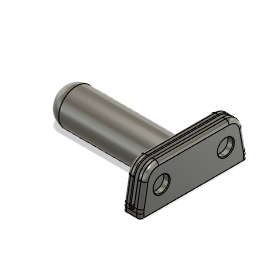
One Piece Handle v3 (Autodesk Fusion 360 design; units mm, degrees)
Autodesk Fusion 360 part; units mm, degrees
note: some values were not read from the file. Chosen so that the rebuilt part matches the saved one: which pieces of a blend or face edit are solid. Set by a fixed rule: which sketch regions a step uses.
sketch "Sketch1" plane through (0, 0, 0) normal (1, 0, 0) x (0, 0, -1)
  line L0 (-37.5, 0) -> (-33.0918, 25)
  line L1 (-33.0918, 25) -> (33.0918, 25)
  line L2 (33.0918, 25) -> (37.5, 0)
  line L3 (37.5, 0) -> (-37.5, 0)
  line L4 (0, 0) -> (0, 25) construction
  dimension "d2" = 75
  dimension "d3" = 80
  dimension "d5" = 100
  dimension "d6" = 25
  constraint horizontal L1
  constraint parallel L1 L3
  constraint coincident L4.start origin
  constraint midpoint L1 L4.end
  constraint vertical L4
  constraint coincident L4.start L3
  measures "d2" distance of L0.start L2.end
  measures "d3" angle of L2 L3
  measures "d5" angle of L0 L3
  measures "d6" distance of L1 L3
extrude "Extrude1" add sketch "Sketch1" along normal blind 5 from surface at 1.125 makes body 1
extrude "Extrude2" add sketch "Sketch1" against normal blind 5 from surface at -1.125 separate body makes body 2
sketch "Sketch2" plane through (0, 0, 0) normal (0, -1, 0) x (1, 0, 0)
  line L0 (1.125, 37.5) -> (1.125, -37.5)
  line L1 (1.125, -37.5) -> (6.125, -37.5)
  line L2 (6.125, -37.5) -> (6.125, 37.5)
  line L3 (6.125, 37.5) -> (1.125, 37.5)
  line L4 (6.125, 37.5) -> (-6.125, 37.5)
  line L5 (-6.125, 37.5) -> (-6.125, -37.5)
  line L6 (-6.125, -37.5) -> (6.125, -37.5)
  line L7 (6.125, -37.5) -> (6.125, 37.5)
  dimension "d13" = 12.25
  dimension "d14" = 75
  constraint horizontal L4
  constraint vertical L5
  constraint horizontal L6
  constraint vertical L7
  constraint coincident L2.end L3.start
  measures "d13" distance of L2.end L4.end
  measures "d14" distance of L2.end L1.end
extrude "Extrude3" add sketch "Sketch2" along normal blind 5 bodies 1 2
sketch "Sketch3" plane through (-6.125, 0, 0) normal (-1, 0, 0) x (0, 0, 1)
  line L0 (-33.0918, 25) -> (-37.5, 0)
  line L1 (-37.5, 0) -> (-37.5, -5)
  line L2 (-37.5, -5) -> (37.5, -5)
  line L3 (37.5, -5) -> (37.5, 0)
  line L4 (37.5, 0) -> (33.0918, 25)
  line L5 (33.0918, 25) -> (-33.0918, 25)
  line L6 (0, -5) -> (0, 5) construction
  circle A0 centre (0, 5) radius 12.5
  dimension "d17" = 25
  dimension "d18" = 10
  constraint midpoint L2 L6.start
  constraint perpendicular L2 L6
  constraint coincident L6.end A0.centre
  measures "d17" diameter of A0
  measures "d18" distance of L6.start L6.end
extrude "Extrude4" add sketch "Sketch3" along normal blind 80 contours L2 A0 picked at (0.0683, 3.2087) bodies 1
fillet "Fillet1" radius 10 1 edges at (-86.125, 17.5, 0) on bodies 1
fillet "Fillet2" radius 10 4 edges at (3.625, 25, 33.0918) (-3.625, 25, 33.0918) (-3.625, 25, -33.0918) (3.625, 25, -33.0918) on bodies 1
fillet "Fillet3" radius 15 4 edges at (3.625, 0, 37.5) (-3.625, 0, 37.5) (-3.625, 0, -37.5) (3.625, 0, -37.5) on bodies 1
fillet "Fillet4" radius 2.5 18 edges at (-6.125, -3.1562, -37.5) (-6.125, -0.005, -37.4429) (-6.125, 9.0144, -35.9105) (-6.125, 22.6604, -31.1287) (-6.125, 25, 0) (-6.125, 22.6604, 31.1287) (-6.125, 9.0144, 35.9105) (-6.125, -0.005, 37.4429) (-6.125, -3.1562, 37.5) (6.125, -3.1562, 37.5) (6.125, -0.005, 37.4429) (6.125, 9.0144, 35.9105) (6.125, 22.6604, 31.1287) (6.125, 25, 0) (6.125, 22.6604, -31.1287) (6.125, 9.0144, -35.9105) (6.125, -0.005, -37.4429) (6.125, -3.1562, -37.5) on bodies 1
chamfer "Chamfer1" distance 1 angle 45 12 edges at (-41.125, -5, 7.5) (-82.7394, -5, 0) (-41.125, -5, -7.5) (-6.125, -5, 21.25) (-6.125, -5, -21.25) (-5.3928, -5, -36.7678) (0, -5, -37.5) (5.3928, -5, -36.7678) (6.125, -5, 0) (5.3928, -5, 36.7678) (0, -5, 37.5) (-5.3928, -5, 36.7678) on bodies 1
sketch "Sketch4" plane through (-6.125, 0, 0) normal (-1, 0, 0) x (0, 0, 1)
  line L0 (8.6747, -4) -> (35, -4)
  line L1 (35, -4) -> (35, -1.3123)
  arc A0 (35, -1.3123) -> (34.8101, 0.8583) centre (22.5, -1.3123) ccw
  line L2 (34.8101, 0.8583) -> (32.0869, 16.3024)
  arc A1 (32.0869, 16.3024) -> (24.7008, 22.5) centre (24.7008, 15) ccw
  line L3 (24.7008, 22.5) -> (-24.7008, 22.5)
  arc A2 (-24.7008, 22.5) -> (-32.0869, 16.3024) centre (-24.7008, 15) ccw
  line L4 (-32.0869, 16.3024) -> (-34.8101, 0.8583)
  arc A3 (-34.8101, 0.8583) -> (-35, -1.3123) centre (-22.5, -1.3123) ccw
  line L5 (-35, -1.3123) -> (-35, -4)
  line L6 (-35, -4) -> (-8.6747, -4)
  arc A4 (8.6747, -4) -> (-8.6747, -4) centre (0, 5) ccw
  circle A5 centre (-22.5, 10) radius 5.5
  circle A6 centre (22.5, 10) radius 5.5
  dimension "d30" = 11
  dimension "d31" = 11
  dimension "d32" = 45
  dimension "d33" = 10
  dimension "d34" = 22.5
  constraint horizontal A5.centre A6.centre
  measures "d30" diameter of A5
  measures "d31" diameter of A6
  measures "d32" horizontal distance of A5.centre A6.centre
  measures "d33" vertical distance of origin A5.centre
  measures "d34" horizontal distance of origin A5.centre
extrude "Extrude5" cut sketch "Sketch4" against normal blind 4 contours A5 | A6 bodies 1
chamfer "Chamfer2" distance 0.5 angle 45 2 edges at (-6.125, 11.9889, 17.3722) (-6.125, 11.9889, -27.6278) on bodies 1
mirror "Mirror1" about plane through (0, 0, 0) normal (1, 0, 0) of "Extrude5", "Chamfer2"
fillet "Fillet5" radius 0.5 2 edges at (-1.125, 0, 0) (1.125, 0, 0) on bodies 1
fillet "Fillet6" radius 0.5 20 edges at (-1.125, 9.0144, -35.9105) (-1.125, 0.897, -37.3364) (-0.9791, 0.147, -37.4288) (0, 0, -37.4425) (0.9791, 0.147, -37.4288) (1.125, 0.897, -37.3364) (1.125, 9.0144, -35.9105) (1.125, 22.6604, -31.1287) (1.125, 25, 0) (1.125, 22.6604, 31.1287) (1.125, 9.0144, 35.9105) (1.125, 0.897, 37.3364) (0.9791, 0.147, 37.4288) (0, 0, 37.4425) (-0.9791, 0.147, 37.4288) (-1.125, 0.897, 37.3364) (-1.125, 9.0144, 35.9105) (-1.125, 22.6604, 31.1287) (-1.125, 25, 0) (-1.125, 22.6604, -31.1287) on bodies 1
equation "d7 = ( 2.25 / 2 ) * 1 mm"
equation "d10 = ( -2.25 / 2 ) * 1 mm"
